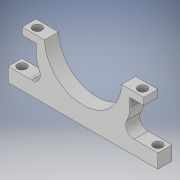
# Autodesk Inventor part: REAL MOTOR MOUNT 2.75 BOTTOM
Saved by Autodesk Inventor 2019 (Build 230136000, 136)
## iProperties
Created: 2018-01-16
Part Number: REAL MOTOR MOUNT 2.75 BOTTOM
Material: Generic
Document SubType Name: Modeling
Designer: Administrator
Density: 1 g/cm^3
Appearance: Default
Author: Administrator
Autodesk Inventor part; units mm, degrees
ref_plane "YZ Plane" through (0, 0, 0) normal (1, 0, 0) x (0, 1, 0)
ref_plane "XZ Plane" through (0, 0, 0) normal (0, 1, 0) x (-1, 0, 0)
ref_plane "XY Plane" through (0, 0, 0) normal (0, 0, 1) x (1, 0, 0)
sketch "Sketch1" plane through (0, 0, 0) normal (0, 0, 1) x (1, 0, 0)
  arc A0 (-39.344, -1.4316) -> (30.4598, -1.4316) centre (-4.4421, -0.1616) ccw
  line L0 (-39.344, -1.4316) -> (-39.3671, -1.4316)
  line L1 (-39.344, -1.4316) -> (-52.044, -1.4316)
  line L2 (30.4598, -1.4316) -> (43.1598, -1.4316)
  arc A1 (-46.964, -22.4724) -> (38.0798, -22.4724) centre (-4.4421, -0.1616) ccw
  line L3 (-4.4421, -48.1813) -> (-4.4421, -51.3563)
  line L4 (-4.4421, -51.3563) -> (-72.364, -51.3563)
  line L5 (-4.4421, -51.3563) -> (63.4798, -51.3563)
  line L6 (-52.044, -1.4316) -> (-59.664, -1.4316)
  line L7 (43.1598, -1.4316) -> (50.7798, -1.4316)
  line L8 (30.4598, -1.4316) -> (38.0798, -1.4316)
  line L9 (38.0798, -1.4316) -> (38.0798, -22.4724)
  line L10 (-39.344, -1.4316) -> (-45.694, -1.4316)
  line L11 (-39.344, -1.4316) -> (-46.964, -1.4316)
  line L12 (-46.964, -1.4316) -> (-46.964, -22.4724)
  line L13 (-46.964, -7.7816) -> (-59.664, -7.7816)
  line L14 (-59.664, -7.7816) -> (-59.664, -1.4316)
  line L15 (38.0798, -7.7816) -> (50.7798, -7.7816)
  line L16 (50.7798, -7.7816) -> (50.7798, -1.4316)
  line L17 (-72.364, -51.3563) -> (-72.364, -38.6563)
  line L18 (63.4798, -51.3563) -> (63.4798, -38.6563)
  line L19 (-72.364, -38.6563) -> (-33.1483, -38.6563)
  line L20 (63.4798, -38.6563) -> (24.2642, -38.6563)
  point P0 (0, 0)
  dimension "d0" = 69.85
  dimension "d1" = 12.7
  dimension "d2" = 12.7
  dimension "d3" = 3.175
  dimension "d4" = 7.62
  dimension "d5" = 7.62
  dimension "d6" = 7.62
  dimension "d7" = 7.62
  dimension "d8" = 6.35
  dimension "d9" = 6.35
  dimension "d10" = 12.7
  dimension "d11" = 12.7
  dimension "d12" = 12.7
  dimension "d13" = 12.7
  constraints: 42 end point, 8 horizontal, 7 point on circle, 6 point on line, 5 vertical, 2 centre point, 2 perpendicular, 1 coincident, 1 concentric, 1 midpoint
  measures "d0" diameter of A0
  measures "d1" distance of L8.start L2.end
  measures "d2" distance of L0.start L1.end
  measures "d3" distance of L3.start L5.start
  measures "d4" distance of L1.end L6.end
  measures "d5" distance of L2.end L16.end
  measures "d6" distance of L8.start L8.end
  measures "d7" distance of L0.start L12.start
  measures "d8" distance of L14.start L6.end
  measures "d9" distance of L16.start L16.end
  measures "d10" distance of L5.end L20.start
  measures "d11" distance of L4.end L19.start
  measures "d12" distance between parallel lines of L17 L14
  measures "d13" distance between parallel lines of L18 L16
extrude "Extrusion1" add sketch "Sketch1" along normal blind 12.7
fillet "Fillet1" radius 7.62 2 edges at (24.2642, -38.6563, 6.35) (-33.1483, -38.6563, 6.35)
fillet "Fillet2" radius 25.4 2 edges at (-46.964, -22.4724, 6.35) (38.0798, -22.4724, 6.35)
sketch "Sketch2" plane through (-59.664, -1.4316, 0) normal (0, 1, 0) x (1, 0, 0)
  line L0 (20.32, 0) -> (20.32, -12.7) projected
  line L1 (0, 0) -> (20.32, 0)
  circle A0 centre (7.62, -6.35) radius 4.064
  circle A1 centre (102.8238, -6.35) radius 4.064
  line L2 (90.1238, 0) -> (90.1238, -12.7) projected
  line L3 (-12.7, 0) -> (-12.7, -12.7) projected
  line L4 (-12.7, -12.7) -> (0, -12.7)
  line L5 (0, -12.7) -> (0, 0)
  line L6 (0, 0) -> (-12.7, 0)
  line L7 (-12.7, 0) -> (-12.7, -12.7)
  line L8 (110.4438, 0) -> (110.4438, -12.7) projected
  line L9 (-12.7, 0) -> (123.1438, 0) projected
  line L10 (110.4438, -12.7) -> (123.1438, -12.7)
  line L11 (123.1438, -12.7) -> (123.1438, 0)
  line L12 (123.1438, 0) -> (110.4438, 0)
  line L13 (110.4438, 0) -> (110.4438, -12.7)
  circle A2 centre (-6.35, -6.35) radius 4.064
  circle A3 centre (116.7892, -6.35) radius 4.064
  point P0 (59.664, 0)
  dimension "d18" = 12.7
  dimension "d19" = 8.128
  dimension "d20" = 12.7
  dimension "d21" = 8.128
  dimension "d22" = 8.128
  dimension "d23" = 8.128
  dimension "d28" = 123.1392
  constraints: 18 end point, 4 centre point, 4 parallel, 3 perpendicular, 2 horizontal
  measures "d18" distance from line of L2 A1.centre
  measures "d19" diameter of A1
  measures "d20" distance from line of L0 A0.centre
  measures "d21" diameter of A0
  measures "d22" diameter of A3
  measures "d23" diameter of A2
  measures "d28" distance of A3.centre A2.centre
extrude "Extrusion2" cut sketch "Sketch2" against normal blind 25.4 contours A0 | A1
extrude "Extrusion3" cut sketch "Sketch2" against normal blind 76.2 contours A2 | A3
body "Solid1"
